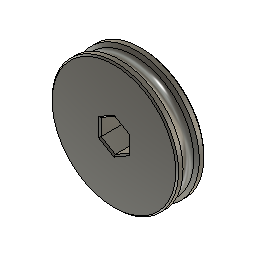
Round Belt Pulley (Autodesk Fusion 360 design; units mm, degrees)
Autodesk Fusion 360 part; units mm, degrees
sketch "Profile" plane through (0, 0, 0) normal (1, 0, 0) x (0, 1, 0)
  line L0 (-6.35, 0) -> (-6.35, 28.575)
  line L1 (-6.35, 28.575) -> (-3.6662, 28.575)
  line L2 (-3.6662, 28.575) -> (-2.7496, 26.9875)
  line L3 (0, 0) -> (0, 28.575) construction
  arc A0 (-2.7496, 26.9875) -> (2.7496, 26.9875) centre (0, 28.575) ccw
  line L4 (0, 0) -> (-6.35, 0)
  line L5 (0, 25.4) -> (2.7496, 25.4) construction
  line L6 (2.7496, 25.4) -> (2.7496, 26.9875) construction
  line L7 (3.6662, 28.575) -> (2.7496, 26.9875)
  line L8 (6.35, 28.575) -> (3.6662, 28.575)
  line L9 (6.35, 0) -> (6.35, 28.575)
  line L10 (0, 0) -> (6.35, 0)
  dimension "d7" = 28.575
  dimension "d9" = 120
  dimension "d10" = 3.175
  dimension "d12" = 6.35
  dimension "d13" = 25.4
  constraint vertical L0
  constraint perpendicular L0 L1
  constraint coincident L3.start L4.start
  constraint vertical L3
  constraint coincident L3.end A0.centre
  constraint horizontal L4
  constraint symmetric L3 L2.end A0.end
  constraint tangent L2 A0
  constraint midpoint A0 L5.start
  constraint tangent A0 L5
  constraint perpendicular L3 L5
  constraint vertical L6
  constraint symmetric L0.start L3 L9.start
  constraint symmetric L0.end L3 L8.start
  constraint symmetric L1.end L3 L7.start
  constraint symmetric L3 L4.start L10.start
  measures "d7" distance of L0.start L0.end
  measures "d9" angle of L1 L2
  measures "d10" radius of A0
  measures "d12" distance of L0.start L3.start
  measures "d13" distance of L4 L5
revolve "Revolve1" add sketch "Profile" angle 360 about axis through (0, 0, 0) along (0, -1, 0)
sketch "Shaft" plane through (0, -6.35, 0) normal (0, -1, 0) x (1, 0, 0)
  line L0 (0, 7.479) -> (-6.477, 3.7395)
  line L1 (-6.477, 3.7395) -> (-6.477, -3.7395)
  line L2 (-6.477, -3.7395) -> (0, -7.479)
  line L3 (0, -7.479) -> (6.477, -3.7395)
  line L4 (6.477, -3.7395) -> (6.477, 3.7395)
  line L5 (6.477, 3.7395) -> (0, 7.479)
  circle A0 centre (0, 0) radius 28.575
  dimension "d15" = 6.477
  constraint vertical L1
  measures "d15" distance of A0.centre L5
extrude "Extrude1" cut sketch "Shaft" against normal through all contours L0 L1 L2 L3 L4 L5
chamfer "Chamfer1" distance 0.635 angle 45 14 edges at (-3.2385, -6.35, 5.6092) (3.2385, -6.35, 5.6092) (6.477, -6.35, 0) (3.2385, -6.35, -5.6092) (-3.2385, -6.35, -5.6092) (-6.477, -6.35, 0) (3.2385, 6.35, 5.6092) (-3.2385, 6.35, 5.6092) (-6.477, 6.35, 0) (-3.2385, 6.35, -5.6092) (3.2385, 6.35, -5.6092) (6.477, 6.35, 0) (-26.6413, -6.35, 10.3332) (-26.6413, 6.35, 10.3332)
equation "PRINTER_TOLERANCE_MED = 0.01 in" comment "Tolerance for printer innacuracy"
equation "PRINTER_OVERHANG = 60 deg" comment "Overhang we can print"
equation "PULLEY_HEX_DIAMETER = 0.5 in" comment "Diameter of hex shaft"
equation "BELT_DIAMETER = 0.25 in" comment "Diameter of the round belt"
equation "PULLEY_BELT_DIAMETER = 2 in" comment "Diameter of pulley where belt contacts it"
equation "PULLEY_OD = PULLEY_BELT_DIAMETER + 0.25 in" comment "OD of Pulley"
equation "d7 = PULLEY_OD / 2"
equation "d9 = 180 deg - PRINTER_OVERHANG"
equation "d10 = BELT_DIAMETER / 2"
equation "PULLEY_WIDTH = 0.5 in" comment "Width of the pulley"
equation "d12 = PULLEY_WIDTH / 2"
equation "d13 = PULLEY_BELT_DIAMETER / 2"
equation "d15 = PULLEY_HEX_DIAMETER / 2 + PRINTER_TOLERANCE_MED / 2"
